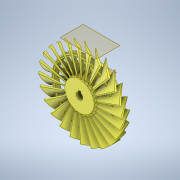
# Autodesk Inventor part: newRotor.24.1.4
Saved by Autodesk Inventor 2021.2 (Build 252289000, 289)
## iProperties
Created: 2021-05-16
Part Number: newRotor.24.1.4
Material: Generic
Document SubType Name: Modeling
Designer: Ryan
Density: 1 g/cm^3
Appearance: Smooth - Yellow
Author: Ryan
## iProperties of the stored document _3DPrint.ipt
Created: 2021-05-23
Part Number: _3DPrint
Material: Generic
Document SubType Name: Modeling
Designer: Ryan
Density: 1 g/cm^3
Appearance: Default
Author: Ryan
Autodesk Inventor part; units mm, degrees
ref_plane "YZ Plane" through (0, 0, 0) normal (1, 0, 0) x (0, 1, 0)
ref_plane "XY Plane" through (0, 0, 0) normal (0, 0, 1) x (1, 0, 0)
sketch "Sketch1" plane through (0, 0, 0) normal (0, 0, 1) x (1, 0, 0)
  circle A0 centre (0, 0) radius 17.78
  dimension "d0" = 35.56
  constraints: 1 centre point, 1 coincident
  measures "d0" diameter of A0
extrude "Extrusion1" add sketch "Sketch1" against normal blind 25.4 draft 11.31
ref_plane "Work Plane1" through (0, 20.32, 0) normal (0, 1, 0) x (-1, 0, 0)
ref_plane "Work Plane2" through (0, 50.8, 0) normal (0, 1, 0) x (-1, 0, 0)
sketch "Sketch5" plane through (0, 20.32, 0) normal (0, 1, 0) x (-1, 0, 0)
  line L0 (17.78, 0) -> (22.86, -25.4) projected
  line L1 (20.32, -12.7) -> (13.268, -12.7)
  line L2 (17.78, 0) -> (-17.78, 0) projected
  line L3 (0, 0) -> (0, -26.8939)
  arc A0 (-0.9632, -0.0899) -> (-1.5903, -1.2672) centre (-1.2978, -0.6673) ccw
  arc A1 (2.9711, -11.9063) -> (-0.9632, -0.0899) centre (-10.1593, -9.7149) ccw
  arc A2 (2.9711, -11.9063) -> (-1.5903, -1.2672) centre (-11.2406, -11.702) ccw
  line L4 (20.32, -12.7) -> (-20.32, -12.7)
  line L5 (-17.78, 0) -> (-22.86, -25.4) projected
  line L6 (3.3558, -11.1125) -> (0, -11.1125)
  point P0 (2.9603, -11.1125)
  point P1 (3.0791, -11.1125)
  point P2 (0, -1.1128)
  point P3 (0, -3.0035)
  dimension "d75" = 0.7937
  dimension "d76" = 1.5875
  constraints: 8 end point, 6 point on circle, 3 centre point, 2 horizontal, 2 midpoint, 1 point on line, 1 vertical
  measures "d75" distance from line of L4 A1.start
  measures "d76" distance between parallel lines of L4 L6
sketch "Sketch6" plane through (0, 50.8, 0) normal (0, 1, 0) x (-1, 0, 0)
  line L0 (17.78, 0) -> (-17.78, 0) projected
  line L1 (-17.78, 0) -> (-22.86, -25.4) projected
  line L2 (22.86, -25.4) -> (-22.86, -25.4) projected
  line L3 (0, -25.4) -> (0, 15.7367)
  arc A0 (1.744, -0.3662) -> (0.5163, -2.4123) centre (1.1254, -1.3864) ccw
  line L4 (-17.78, 0) -> (-22.86, -25.4) projected
  line L5 (-20.32, -12.7) -> (28.4724, -12.7)
  arc A1 (19.366, -11.1125) -> (1.3412, -0.213) centre (-18.9155, -54.0657) ccw
  arc A2 (19.089, -11.1125) -> (0.5163, -2.4123) centre (-20.414, -71.2672) ccw
  line L6 (19.366, -11.1125) -> (19.089, -11.1125)
  point P0 (0, 0)
  dimension "d82" = 1.5875
  constraints: 8 point on circle, 6 end point, 3 centre point, 2 horizontal, 2 midpoint, 1 vertical
  measures "d82" distance between parallel lines of L6 L5
sketch "Sketch8" plane through (0, 0, 0) normal (0, 0, 1) x (1, 0, 0)
  circle A0 centre (0, 0) radius 4
  line L0 (-1.5875, 5.5875) -> (1.5875, 5.5875)
  line L1 (1.5875, 5.5875) -> (1.5875, 2.4125)
  line L2 (1.5875, 2.4125) -> (-1.5875, 2.4125)
  line L3 (-1.5875, 2.4125) -> (-1.5875, 5.5875)
  line L4 (-1.5875, 5.5875) -> (1.5875, 2.4125) construction
  line L5 (1.5875, 5.5875) -> (-1.5875, 2.4125) construction
  point P0 (0, 4)
  point P1 (-1.5875, 3.6715)
  point P2 (1.5875, 3.6715)
  dimension "d39" = 8
  dimension "d40" = 3.175
  dimension "d41" = 3.175
  constraints: 12 end point, 2 midpoint, 2 parallel, 1 coincident, 1 horizontal, 1 perpendicular, 3 other
  measures "d40" distance of L1.end L2.end
  measures "d41" distance of L0.end L1.end
extrude "Extrusion5" cut sketch "Sketch8" against normal through all
sketch "Sketch13" plane through (0, 0, 0) normal (0, 0, 1) x (1, 0, 0)
  circle A0 centre (0, 0) radius 17.78 projected
  circle A1 centre (0, 0) radius 50.0063
  arc A2 (-1.5875, 3.6715) -> (1.5875, 3.6715) centre (0, 0) ccw projected
  circle A3 centre (0, 0) radius 80.6636
  point P0 (9.9902, -14.708)
  point P1 (13.4565, -11.6212)
  dimension "d66" = 100.0125
  constraints: 2 centre point, 2 coincident
  measures "d66" diameter of A1
extrude "Extrusion7" add sketch "Sketch5" against normal blind 5.08 contours A0 A1 L3 A2 | A1 L6 A2 L3
loft "Loft5" add profiles "Sketch6" section 1 edges at (-2.3387, 20.32, -5.1315) (1.8868, 20.32, -0.3536) (-1.6611, 20.32, -5.7387) (-3.0197, 20.32, -11.1125) contours A0 A1 L6 A2 L3 | L3 A0
pattern_circular "Circular Pattern6" count 24 over 360 about axis through (0, 0, 0) along (0, 0, -1) of "Loft5", "Extrusion7"
sketch "Sketch14" plane through (0, 0, 0) normal (1, 0, 0) x (0, 1, 0)
  line L0 (36.83, -3.4925) -> (36.195, -3.4925)
  line L1 (34.925, -4.7625) -> (34.925, -9.8425)
  line L2 (36.195, -11.1125) -> (36.83, -11.1125)
  line L3 (38.1, -9.8425) -> (38.1, -4.7625)
  line L4 (50.8, 5.1345) -> (50.8, -30.4891) projected
  arc A0 (38.1, -4.7625) -> (36.83, -3.4925) centre (36.83, -4.7625) ccw
  arc A1 (36.83, -11.1125) -> (38.1, -9.8425) centre (36.83, -9.8425) ccw
  arc A2 (34.925, -9.8425) -> (36.195, -11.1125) centre (36.195, -9.8425) ccw
  arc A3 (36.195, -3.4925) -> (34.925, -4.7625) centre (36.195, -4.7625) ccw
  line L5 (12.7237, -11.1125) -> (41.9316, -11.1125) projected
  line L6 (0, -30.4891) -> (0, 5.1345) projected
  point P0 (0, 0)
  point P1 (38.1, -3.4925)
  point P2 (34.925, -11.1125)
  point P3 (38.1, -11.1125)
  dimension "d90" = 7.62
  dimension "d91" = 3.175
  dimension "d92" = 12.7
  dimension "d93" = 1.27
  dimension "d94" = 0
  constraints: 8 end point, 8 point on circle, 8 tangent, 6 point on line, 4 centre point, 3 equal radius, 2 parallel, 1 horizontal, 1 perpendicular
  measures "d90" distance of point (38.1, -11.112) point (38.1, -3.492)
  measures "d91" distance of point (34.925, -11.112) point (38.1, -11.112)
  measures "d92" distance between parallel lines of L3 L4
  measures "d93" radius of A0
  measures "d94" distance between parallel lines of L2 L5
revolve "Revolution5" add sketch "Sketch14" angle 360 about axis through (0, 0, -10) along (0, 0, 1)
extrude "Extrusion8" cut sketch "Sketch13" against normal through all contours A3
body "Solid1"
